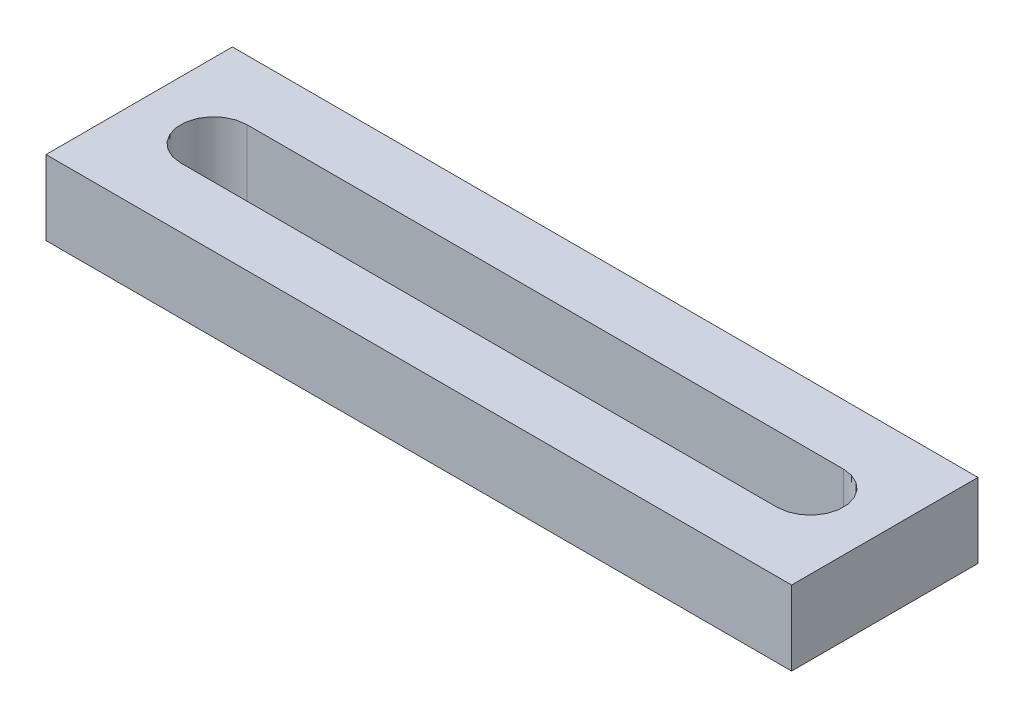
# Autodesk Inventor part: ChipClip
Saved by Autodesk Inventor 2019 (Build 230136000, 136)
## iProperties
Created: 2019-08-13
Part Number: ChipClip
Material: Generic
Document SubType Name: Modeling
Designer: aorfi
Density: 1 g/cm^3
Appearance: Default
Author: aorfi
Autodesk Inventor part; units mm, degrees
ref_plane "YZ Plane" through (0, 0, 0) normal (1, 0, 0) x (0, 1, 0)
ref_plane "XZ Plane" through (0, 0, 0) normal (0, 1, 0) x (-1, 0, 0)
ref_plane "XY Plane" through (0, 0, 0) normal (0, 0, 1) x (1, 0, 0)
sketch "Sketch1" plane through (0, 0, 0) normal (0, 1, 0) x (-1, 0, 0)
  line L0 (10, 2.5) -> (-10, 2.5)
  line L1 (-10, 2.5) -> (-10, -2.5)
  line L2 (-10, -2.5) -> (10, -2.5)
  line L3 (10, -2.5) -> (10, 2.5)
  line L4 (10, 2.5) -> (-10, -2.5) construction
  line L5 (-10, 2.5) -> (10, -2.5) construction
  circle A0 centre (8, 0) radius 0.889
  circle A1 centre (-8, 0) radius 0.889
  line L6 (8, -0.889) -> (-8, -0.889)
  line L7 (8, 0.889) -> (-8, 0.889)
  point P0 (0, 0)
  point P1 (0, 0)
  point P2 (0, 0)
  point P3 (0, 0)
  dimension "d19" = 20
  dimension "d20" = 5
  dimension "d21" = 1.778
  dimension "d22" = 2
  dimension "d23" = 2
  constraints: 16 end point, 4 midpoint, 4 point on circle, 3 parallel, 2 centre point, 2 horizontal, 2 horizontal alignment, 2 tangent, 1 coincident, 1 equal radius, 1 perpendicular
  measures "d19" distance of L1.end L2.end
  measures "d20" distance of L0.end L1.end
  measures "d21" diameter of A0
  measures "d22" distance from line of A0.centre L3
  measures "d23" distance from line of L1 A1.centre
extrude "Extrusion1" add sketch "Sketch1" along normal mid plane 2
body "Solid1"
